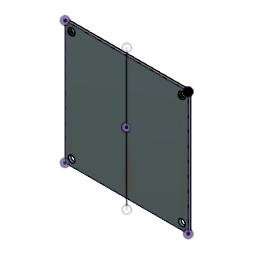
Atlas_SurfaceModule_SM-001 (Autodesk Fusion 360 design; units mm, degrees)
part number: 2026-07-07-10-45-00-715
Autodesk Fusion 360 part; units mm, degrees
sketch "Module Outline" plane through (0, 0, 0) normal (0, 0, 1) x (1, 0, 0)
  line L0 (-120.65, -120.65) -> (120.65, -120.65)
  line L1 (120.65, -120.65) -> (120.65, 120.65)
  line L2 (120.65, 120.65) -> (-120.65, 120.65)
  line L3 (-120.65, 120.65) -> (-120.65, -120.65)
  line L4 (-120.65, -120.65) -> (120.65, 120.65) construction
  line L5 (120.65, -120.65) -> (-120.65, 120.65) construction
  dimension "d17" = 241.3
  dimension "d18" = 241.3
  constraint horizontal L0
  constraint perpendicular L0 L1
  constraint parallel L0 L2
  constraint parallel L1 L3
  constraint coincident L4 origin
  constraint coincident L5 origin
  measures "d17" distance of L0.start L2.end
  measures "d18" distance of L1.end L2.end
extrude "Shelf Plate" add sketch "Module Outline" along normal blind 5.08
sketch "Anchor Locations" plane through (0, 0, 5.08) normal (0, 0, 1) x (1, 0, 0)
  line L0 (-120.65, 120.65) -> (-120.65, -120.65)
  line L1 (-120.65, -120.65) -> (120.65, -120.65)
  line L2 (120.65, -120.65) -> (120.65, 120.65)
  line L3 (120.65, 120.65) -> (-120.65, 120.65)
  line L4 (120.65, 120.65) -> (107.95, 107.95) construction
  line L5 (120.65, -120.65) -> (120.65, 120.65) construction
  line L6 (-120.65, -120.65) -> (120.65, -120.65) construction
  line L7 (-120.65, 120.65) -> (-120.65, -120.65) construction
  line L8 (120.65, 120.65) -> (-120.65, 120.65) construction
  line L9 (0, 134.6139) -> (0, -139.7)
  point P0 (-107.95, 107.95)
  dimension "d22" = 12.7
  dimension "d23" = 12.7
  constraint coincident L2.end L3.start
  constraint perpendicular L1 L9
  constraint vertical origin L9.start
  constraint symmetric L4.end L9 P0
  measures "d22" distance of L2 L4.end
  measures "d23" distance of L3 L4.end
sketch "Socket Geometry" plane through (0, 0, 5.08) normal (0, 0, 1) x (1, 0, 0)
  line L0 (-120.65, 120.65) -> (-120.65, -120.65)
  line L1 (-120.65, -120.65) -> (120.65, -120.65)
  line L2 (120.65, -120.65) -> (120.65, 120.65)
  line L3 (120.65, 120.65) -> (-120.65, 120.65)
  circle A0 centre (107.95, 107.95) radius 6.5532
  line L4 (0, 127) -> (0, -127)
  circle A1 centre (-107.95, 107.95) radius 6.5532
  line L5 (-130.6691, 0) -> (143.6907, 0)
  circle A2 centre (107.95, -107.95) radius 6.5532
  circle A3 centre (-107.95, -107.95) radius 6.5532
  point P0 (107.95, 107.95)
  point P1 (-101.6, 101.6)
  point P2 (-101.6, -101.6)
  point P3 (101.6, -101.6)
  dimension "d28" = 13.1064
  constraint coincident P0 A0.centre
  constraint symmetric A0 L4 A1
  constraint symmetric A0 L5 A2
  constraint symmetric A1 L5 A3
  measures "d28" diameter of A0
extrude "Socket Cut" cut sketch "Socket Geometry" against normal blind 7.62 contours A0 | A1 | A2 | A3
equation "shelfLength = 12 in"
equation "shelfDepth = 8 in"
equation "shelfThickness = 0.20 in"
equation "lipHeight = 1 in"
equation "cornerRadius = 0.5 in"
equation "clearance = 0.008 in"
equation "tileWidth = 9.5 in"
equation "tileDepth = 9.5 in"
equation "tileThickness = 0.2 in"
equation "columnSocketDiameter = 0.75 in"
equation "columnDiameter = 0.7 in"
equation "socketInset = 0.5 in"
equation "socketDepth = 0.3 in"
equation "socketWall = 0.12 in"
equation "filletSmall = 0.06 in"
equation "filletMedium = 0.12 in"
equation "d17 = tileWidth"
equation "d18 = tileDepth"
equation "d19 = shelfThickness"
equation "anchorOffset = 0.5 in"
equation "d22 = anchorOffset"
equation "d23 = anchorOffset"
equation "pinDiameter = 0.5 in"
equation "socketDiameter = pinDiameter + ( 2 * clearance )"
equation "d28 = socketDiameter"
equation "d29 = -socketDepth"
named bodies: "Surface Module"
